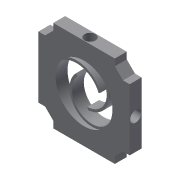
# Autodesk Inventor part: 50_Cube_Insert_Thorlabs
Saved by Autodesk Inventor 2019 (Build 230136000, 136)
## iProperties
Created: 2019-07-01
Part Number: 50_Cube_Insert_Thorlabs
Material: Generic
Document SubType Name: Modeling
Designer: diederichbenedict
Density: 1 g/cm^3
Appearance: Default
Author: diederichbenedict
Autodesk Inventor part; units mm, degrees
ref_plane "YZ Plane" through (0, 0, 0) normal (1, 0, 0) x (0, 1, 0)
ref_plane "Work Plane1" through (0, 0, 10) normal (0, 0, 1) x (1, 0, 0)
sketch "Sketch1" plane through (0, 0, 10) normal (0, 0, 1) x (1, 0, 0)
  line L0 (-4.0299, -0.3538) -> (-2.2322, 1.4439) construction
  arc A0 (-1.4439, 2.2322) -> (-2.2322, 1.4439) centre (-0.9299, 0.9299) ccw construction
  line L1 (-1.4439, 2.2322) -> (0.3538, 4.0299) construction
  line L2 (-37.8299, 42.2137) -> (-37.8299, 45.8299) construction
  line L3 (-37.8299, 45.8299) -> (-4.0299, 45.8299) construction
  line L4 (-4.0299, 45.8299) -> (-4.0299, 42.2137) construction
  line L5 (-4.0299, 4.0299) -> (0.3538, 4.0299) projected
  line L6 (-20.9299, 58.9723) -> (17.1124, 20.9299) construction
  line L7 (17.1124, 20.9299) -> (-20.9299, -17.1124) construction
  line L8 (-20.9299, -17.1124) -> (-58.9723, 20.9299) construction
  line L9 (-58.9723, 20.9299) -> (-20.9299, 58.9723) construction
  line L10 (-20.9299, 58.9723) -> (-20.9299, -17.1124) construction
  line L11 (17.1124, 20.9299) -> (-58.9723, 20.9299) construction
  line L12 (-20.9299, 58.9723) -> (32.8701, 58.9723) construction
  line L13 (-43.4299, 43.4299) -> (1.5701, 43.4299) construction
  line L14 (1.5701, 43.4299) -> (1.5701, -1.5701) construction
  line L15 (1.5701, -1.5701) -> (-43.4299, -1.5701) construction
  line L16 (-43.4299, -1.5701) -> (-43.4299, 43.4299) construction
  line L17 (-43.4299, 43.4299) -> (1.5701, -1.5701) construction
  line L18 (1.5701, 43.4299) -> (-43.4299, -1.5701) construction
  line L19 (-43.4299, 5.3876) -> (-43.4299, 36.4723)
  line L20 (-43.4299, 36.4723) -> (-36.4723, 43.4299)
  line L21 (-36.4723, 43.4299) -> (-5.3876, 43.4299)
  line L22 (-5.3876, 43.4299) -> (1.5701, 36.4723)
  line L23 (1.5701, 36.4723) -> (1.5701, 5.3876)
  line L24 (1.5701, 5.3876) -> (-5.3876, -1.5701)
  line L25 (-5.3876, -1.5701) -> (-36.4723, -1.5701)
  line L26 (-36.4723, -1.5701) -> (-43.4299, 5.3876)
  line L27 (-4.0299, 42.2137) -> (-37.8299, 42.2137) projected
  line L28 (-4.0299, -0.3538) -> (-4.0299, 4.0299) projected
  circle A1 centre (-20.9299, 20.9299) radius 13.3985
  circle A2 centre (-20.9299, 20.9299) radius 15.4895
  point P0 (-37.8299, 4.0299)
  dimension "d18" = 53.8
  dimension "d19" = 45
  dimension "d20" = 53.8
  dimension "d21" = 45
  dimension "d22" = 45
  dimension "d30" = 26.797
  dimension "d36" = 30.979
  constraints: 42 end point, 15 point on line, 4 parallel, 3 midpoint, 3 perpendicular, 2 centre point, 2 coincident, 2 horizontal, 1 equal length
  measures "d18" distance of L6.start L6.end
  measures "d19" angle of L6 L12
  measures "d20" distance of L6.end L7.end
  measures "d21" distance of L14.end L15.end
  measures "d22" distance of L13.end L14.end
  measures "d30" diameter of A1
  measures "d36" diameter of A2
extrude "Extrusion1" add sketch "Sketch1" along normal blind 6.5 contours L28 L24 L25 L26 L19 L20 L27 L22 L23 L5 | L5 L24 L28 | L27 L20 L21 L22 | A1 | A2
ref_plane "Work Plane2" through (-40.9959, 0.8639, 22.2359) normal (0, 0, 1) x (1, 0, 0)
sketch "Sketch3" plane through (0, 0, 10) normal (0, 0, -1) x (-1, 0, 0)
  line L0 (37.8299, -0.4701) -> (37.8299, 4.0299) construction
  line L1 (4.0299, 4.0299) -> (4.0299, -0.4701) construction
  line L2 (37.8299, -0.4701) -> (37.8299, 1.1886) construction
  line L3 (4.0299, -3.9701) -> (4.0299, -0.3538) construction
  line L4 (45.8299, 4.0299) -> (42.2137, 4.0299) construction
  line L5 (-0.3538, 4.0299) -> (-3.9701, 4.0299) construction
  line L6 (-3.9701, 37.8299) -> (-0.3538, 37.8299) construction
  line L7 (4.0299, 42.2137) -> (4.0299, 45.8299) construction
  line L8 (37.8299, 45.8299) -> (37.8299, 42.2137) construction
  line L9 (42.2137, 37.8299) -> (45.8299, 37.8299) construction
  line L10 (37.8299, 37.7299) -> (45.8299, 37.7299)
  line L11 (45.8299, 37.7299) -> (45.8299, 4.1299)
  line L12 (45.8299, 4.1299) -> (37.8299, 4.1299)
  line L13 (37.8299, 4.1299) -> (37.8299, 37.7299)
  line L14 (37.7299, 4.0299) -> (4.1299, 4.0299)
  line L15 (4.1299, 4.0299) -> (4.1299, -3.9701)
  line L16 (4.1299, -3.9701) -> (37.7299, -3.9701)
  line L17 (37.7299, -3.9701) -> (37.7299, 4.0299)
  line L18 (4.0299, 4.1299) -> (-3.9701, 4.1299)
  line L19 (-3.9701, 4.1299) -> (-3.9701, 37.7299)
  line L20 (-3.9701, 37.7299) -> (4.0299, 37.7299)
  line L21 (4.0299, 37.7299) -> (4.0299, 4.1299)
  line L22 (4.1299, 37.8299) -> (37.7299, 37.8299)
  line L23 (37.7299, 37.8299) -> (37.7299, 45.8299)
  line L24 (37.7299, 45.8299) -> (4.1299, 45.8299)
  line L25 (4.1299, 45.8299) -> (4.1299, 37.8299)
  point P0 (0, 0)
  dimension "d23" = 0.1
  dimension "d24" = 0.1
  dimension "d25" = 0.1
  dimension "d26" = 0.1
  dimension "d27" = 0.1
  constraints: 32 end point, 8 parallel, 4 horizontal, 4 perpendicular, 3 point on line
  measures "d23" distance between parallel lines of L8 L23
  measures "d24" distance between parallel lines of L7 L25
  measures "d25" distance between parallel lines of L6 L20
  measures "d26" distance between parallel lines of L5 L18
  measures "d27" distance between parallel lines of L1 L15
extrude "Extrusion3" add sketch "Sketch3" against normal up to surface (6.5 mm away)
sketch "Sketch6" plane through (0, 0, 16.5) normal (0, 0, 1) x (1, 0, 0)
  circle A0 centre (-20.9299, 20.9299) radius 15.4895
  circle A1 centre (-20.9299, 20.9299) radius 13.3985
  line L0 (-45.8299, 4.1299) -> (-45.8299, 37.7299) projected
  line L1 (-4.1299, -3.9701) -> (-37.7299, -3.9701) projected
  line L2 (-37.7299, 45.8299) -> (-4.1299, 45.8299) projected
  point P0 (0, 0)
  point P1 (-45.8299, 20.9299)
  point P2 (-20.9299, -3.9701)
  point P3 (-20.9299, 45.8299)
  dimension "d37" = 26.797
  dimension "d38" = 30.979
  constraints: 3 midpoint, 2 centre point, 2 vertical alignment, 1 coincident, 1 horizontal alignment
  measures "d37" diameter of A1
  measures "d38" diameter of A0
extrude "Extrusion5" cut sketch "Sketch6" against normal blind 12 contours A0 | A1
sketch "Sketch7" plane through (0, 0, 16.5) normal (0, 0, 1) x (1, 0, 0)
  arc A0 (-12.9538, 25.0869) -> (-28.6747, 7.5156) centre (-25.0755, 20.1138) ccw
  arc A1 (-11.8561, 25.8297) -> (-29.5384, 33.807) centre (-25.0755, 20.1138) ccw
  line L0 (-11.8561, 25.8297) -> (-12.9538, 25.0869)
  arc A2 (-29.5384, 33.807) -> (-28.6747, 7.5156) centre (-20.9299, 20.9299) ccw
  arc A3 (-19.1989, 15.4337) -> (-10.0534, 31.9583) centre (-19.562, 26.4277) ccw
  arc A4 (-7.4473, 28.5552) -> (-10.0534, 31.9583) centre (-19.6452, 21.9138) ccw
  line L1 (-19.4299, 22.4299) -> (-3.5175, 22.4299) construction
  arc A5 (-25.3758, 28.221) -> (-12.1653, 8.1586) centre (-16.5552, 19.6486) ccw
  circle A6 centre (-20.9299, 20.9299) radius 15.4895 construction
  arc A7 (-12.4299, 22.4299) -> (-19.1989, 15.4337) centre (-19.4299, 22.4299) ccw construction
  line L2 (-25.3758, 28.221) -> (-24.4607, 27.2973)
  arc A8 (-24.4607, 27.2973) -> (-6.8601, 14.452) centre (-16.5552, 19.6486) ccw
  circle A9 centre (-20.9299, 20.9299) radius 15.4895 construction
  line L3 (3.9701, 4.1299) -> (0.3124, 4.1299) construction
  line L4 (3.9701, 37.7299) -> (3.9701, 4.1299) construction
  line L5 (0.3124, 37.7299) -> (3.9701, 37.7299) construction
  line L6 (0.3124, 37.7299) -> (-4.1299, 42.1723) construction
  line L7 (-4.1299, 45.8299) -> (-4.1299, 42.1723) construction
  line L8 (-37.7299, 45.8299) -> (-4.1299, 45.8299) construction
  line L9 (-37.7299, 42.1723) -> (-37.7299, 45.8299) construction
  line L10 (-37.7299, 42.1723) -> (-42.1723, 37.7299) construction
  line L11 (-45.8299, 37.7299) -> (-42.1723, 37.7299) construction
  line L12 (-45.8299, 4.1299) -> (-45.8299, 37.7299) construction
  line L13 (-42.1723, 4.1299) -> (-45.8299, 4.1299) construction
  line L14 (-42.1723, 4.1299) -> (-37.7299, -0.3124) construction
  line L15 (-37.7299, -3.9701) -> (-37.7299, -0.3124) construction
  line L16 (-4.1299, -3.9701) -> (-37.7299, -3.9701) construction
  line L17 (-4.1299, -0.3124) -> (-4.1299, -3.9701) construction
  line L18 (-4.1299, -0.3124) -> (0.3124, 4.1299) construction
  line L19 (-19.1989, 15.4337) -> (-18.7812, 14.1526) construction
  arc A10 (-19.1989, 15.4337) -> (-12.4299, 22.4299) centre (-19.4299, 22.4299) ccw construction
  arc A11 (-18.7812, 14.1526) -> (-7.4473, 28.5552) centre (-19.562, 26.4277) ccw
  line L20 (-19.1989, 15.4337) -> (-18.7812, 14.1526) construction
  line L21 (-18.7812, 14.1526) -> (-19.1989, 15.4337)
  arc A12 (-12.1653, 8.1586) -> (-6.8601, 14.452) centre (-13.2455, 14.452) ccw
  line L22 (-28.6747, 7.5156) -> (-20.9299, 20.9299) construction
  line L23 (-20.9299, 20.9299) -> (-5.6794, 18.2195) construction
  line L24 (-6.8601, 14.452) -> (-13.2455, 14.452) construction
  circle A13 centre (-20.9299, 20.9299) radius 15.4895 projected
  point P0 (0, 0)
  point P1 (-17.9152, 11.0615)
  point P2 (-33.1816, 30.4073)
  dimension "d58" = 1.3
  dimension "d60" = 1.3
  dimension "d63" = 1.3
  dimension "d78" = 1.5
  dimension "d79" = 1.5
  dimension "d81" = 11
  dimension "d83" = 11
  dimension "d86" = 7
  dimension "d90" = 0
  dimension "d91" = 120
  constraints: 33 point on circle, 18 end point, 11 centre point, 6 coincident, 3 tangent, 1 collinear, 1 horizontal, 1 point on line, 3 other
  measures "d58" radial gap between concentric circles of A1 A0
  measures "d60" radial gap between concentric circles of A5 A8
  measures "d63" radial gap between concentric circles of A11 A3
  measures "d78" horizontal distance of L1.start A6.centre
  measures "d79" horizontal distance of A6.centre A7.centre
  measures "d81" radius of A3
  measures "d83" radius of A8
  measures "d86" radius of A7
  measures "d90" angle of L8 L24
  measures "d91" angle of L24 L22
extrude "Extrusion6" add sketch "Sketch7" against normal up to surface (6.5 mm away) contours A0 A2 A1 L0 | A5 L2 A8 A13 | A13 A11 L21 A3 | A4 A13
sketch "Sketch8" plane through (-37.7299, 45.8299, 10) normal (0, 1, 0) x (1, 0, 0)
  line L0 (0, 0) -> (33.6, 0) projected
  line L1 (0, -6.5) -> (33.6, -6.5) projected
  line L2 (33.6, 0) -> (33.6, -6.5) projected
  line L3 (0, 0) -> (0, -6.5) projected
  point P0 (37.7299, 10)
  point P1 (16.8, -3.25)
  point P2 (16.8, 0)
  point P3 (16.8, -6.5)
  point P4 (33.6, -3.25)
  point P5 (0, -3.25)
  constraints: 4 midpoint, 2 horizontal alignment, 2 vertical alignment
hole "Hole1" at (-20.9299, 45.8299, 13.25) direction (0, -1, 0) diameter 2.9 depth 11 tip angle 118 counterbore diameter 6 counterbore depth 6
sketch "Sketch9" plane through (3.9701, 4.1299, 10) normal (1, 0, 0) x (0, 0, -1)
  line L0 (0, 0) -> (0, 33.6) projected
  line L1 (-6.5, 33.6) -> (-6.5, 0) projected
  line L2 (0, 33.6) -> (-6.5, 33.6) projected
  line L3 (0, 0) -> (-6.5, 0) projected
  point P0 (10, -4.1299)
  point P1 (-3.25, 16.8)
  point P2 (0, 16.8)
  point P3 (-6.5, 16.8)
  point P4 (-3.25, 33.6)
  point P5 (-3.25, 0)
  constraints: 4 midpoint, 2 horizontal alignment, 2 vertical alignment
hole "Hole2" at (3.9701, 20.9299, 13.25) direction (-1, 0, 0) diameter 2.9 depth 11 tip angle 118 counterbore diameter 6 counterbore depth 6
body "Solid1"
